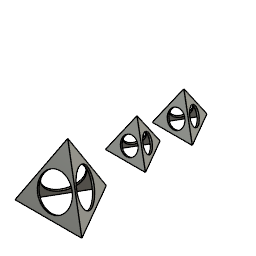
15_DAY- Painter's Tripod (Autodesk Fusion 360 design; units mm, degrees)
part number: 2026-01-01-13-45-42-633
part number: 2026-01-01-14-03-48-325
part number: 2026-01-01-15-44-14-888
part number: 2026-01-01-15-45-19-791
Autodesk Fusion 360 part; units mm, degrees
sketch "Sketch1" plane through (0, 0, 0) normal (0, 1, 0) x (1, 0, 0) in component "60mm Painter's Tripod"
  line L0 (0, 0) -> (30, 51.9615)
  line L1 (30, 51.9615) -> (60, 0)
  line L2 (60, 0) -> (0, 0)
  dimension "d1" = 60
  constraint coincident L0.start L2.end
  constraint horizontal L2
  constraint equal L0 L2
  constraint equal L0 L1
  measures "d1" distance of L0.start L0.end
ref_plane "WorkPlane1" through (30, 50, -25.9808) normal (0, 1, 0) x (1, 0, 0) in component "60mm Painter's Tripod"
sketch "Sketch2" plane through (0, 50, 0) normal (0, 1, 0) x (1, 0, 0) in component "60mm Painter's Tripod"
  line L0 (0, 0) -> (30, 51.9615)
  line L1 (60, 0) -> (0, 0)
  line L2 (30, 51.9615) -> (60, 0)
  line L3 (30, 51.9615) -> (30, 0) construction
  line L4 (0, 0) -> (45, 25.9808) construction
  point P0 (30, 17.3205)
  constraint coincident L0.end L2.start
  constraint midpoint L1 L3.end
  constraint coincident L0.start L1.end
  constraint midpoint L2 L4.end
  constraint coincident L4 P0
  constraint coincident L3 P0
loft "Loft1" add profiles "Sketch1" section 1 section 2 point at (30, 50, -17.3205) makes body 1 in component "60mm Painter's Tripod"
shell "Shell1" thickness 2.5 removed faces 1 at (30, 0, -17.3205) on bodies 1 in component "60mm Painter's Tripod"
sketch "Sketch3" plane through (0, 0, 0) normal (0, 0.327327, 0.944911) x (1, 0, 0) in component "60mm Painter's Tripod"
  line L0 (0, 0) -> (60, 0)
  line L1 (60, 0) -> (30, 52.915)
  line L2 (30, 52.915) -> (0, 0)
  line L3 (30, 52.915) -> (30, 0) construction
  line L4 (0, 0) -> (45, 26.4575) construction
  circle A0 centre (30, 17.6383) radius 12.5
  dimension "d4" = 25
  constraint coincident L1.end L2.start
  constraint midpoint L0 L3.end
  constraint coincident L0.start L2.end
  constraint midpoint L1 L4.end
  constraint coincident L4 A0.centre
  constraint coincident L3 A0.centre
  measures "d4" diameter of A0
extrude "Extrude1" cut sketch "Sketch3" against normal blind 2.5 contours A0 bodies 1 in component "60mm Painter's Tripod"
pattern_circular "C-Pattern1" count 3 over 360 about axis through (30, 75, -17.3205) along (0, -1, 0) of "Extrude1" in component "60mm Painter's Tripod"
sketch "Sketch1 (2)" plane through (0, 0, 0) normal (0, 1, 0) x (1, 0, 0) in component "60mm Painter's Tripod (1)"
  line L0 (0, 0) -> (30, 51.9615)
  line L1 (30, 51.9615) -> (60, 0)
  line L2 (60, 0) -> (0, 0)
  dimension "d1_1" = 60
  constraint coincident L0.start L2.end
  constraint horizontal L2
  constraint equal L0 L2
  constraint equal L0 L1
  measures "d1_1" distance of L0.start L0.end
ref_plane "WorkPlane1" through (30, 50, -25.9808) normal (0, 1, 0) x (1, 0, 0) in component "60mm Painter's Tripod (1)"
sketch "Sketch2 (2)" plane through (0, 50, 0) normal (0, 1, 0) x (1, 0, 0) in component "60mm Painter's Tripod (1)"
  line L0 (0, 0) -> (30, 51.9615)
  line L1 (60, 0) -> (0, 0)
  line L2 (30, 51.9615) -> (60, 0)
  line L3 (30, 51.9615) -> (30, 0) construction
  line L4 (0, 0) -> (45, 25.9808) construction
  point P0 (30, 17.3205)
  constraint coincident L0.end L2.start
  constraint midpoint L1 L3.end
  constraint coincident L0.start L1.end
  constraint midpoint L2 L4.end
  constraint coincident L4 P0
  constraint coincident L3 P0
loft "Loft1'" add profiles "Sketch1 (2)" section 1 section 2 point at (30, 50, -17.3205) separate body makes body 2 in component "60mm Painter's Tripod (1)"
shell "Shell1'" thickness 2.5 removed faces 1 at (30, 0, -17.3205) on bodies 2 in component "60mm Painter's Tripod (1)"
sketch "Sketch3 (2)" plane through (0, 0, 0) normal (0, 0.327327, 0.944911) x (1, 0, 0) in component "60mm Painter's Tripod (1)"
  line L0 (0, 0) -> (60, 0)
  line L1 (60, 0) -> (30, 52.915)
  line L2 (30, 52.915) -> (0, 0)
  line L3 (30, 52.915) -> (30, 0) construction
  line L4 (0, 0) -> (45, 26.4575) construction
  circle A0 centre (30, 17.6383) radius 12.5
  dimension "d4_1" = 25
  constraint coincident L1.end L2.start
  constraint midpoint L0 L3.end
  constraint coincident L0.start L2.end
  constraint midpoint L1 L4.end
  constraint coincident L4 A0.centre
  constraint coincident L3 A0.centre
  measures "d4_1" diameter of A0
extrude "Extrude1'" cut sketch "Sketch3 (2)" against normal blind 2.5 contours A0 bodies 2 in component "60mm Painter's Tripod (1)"
pattern_circular "C-Pattern1'" count 3 over 360 about axis through (30, 75, -17.3205) along (0, -1, 0) of "Extrude1'" in component "60mm Painter's Tripod (1)"
sketch "Sketch1 (3)" plane through (0, 0, 0) normal (0, 1, 0) x (1, 0, 0) in component "60mm Painter's Tripod NEW"
  line L0 (0, 0) -> (50, 86.6025)
  line L1 (50, 86.6025) -> (100, 0)
  line L2 (100, 0) -> (0, 0)
  dimension "d1_2" = 100
  constraint coincident L0.start L2.end
  constraint horizontal L2
  constraint equal L0 L2
  constraint equal L0 L1
  measures "d1_2" distance of L0.start L0.end
ref_plane "WorkPlane1" through (50, 90, -43.3013) normal (0, 1, 0) x (1, 0, 0) in component "60mm Painter's Tripod NEW"
sketch "Sketch2 (3)" plane through (0, 90, 0) normal (0, 1, 0) x (1, 0, 0) in component "60mm Painter's Tripod NEW"
  line L0 (0, 0) -> (50, 86.6025)
  line L1 (100, 0) -> (0, 0)
  line L2 (50, 86.6025) -> (100, 0)
  line L3 (50, 86.6025) -> (50, 0) construction
  line L4 (0, 0) -> (75, 43.3013) construction
  point P0 (50, 28.8675)
  constraint coincident L0.end L2.start
  constraint midpoint L1 L3.end
  constraint coincident L0.start L1.end
  constraint midpoint L2 L4.end
  constraint coincident L4 P0
  constraint coincident L3 P0
loft "Loft1''" add profiles "Sketch1 (3)" section 1 section 2 point at (50, 90, -28.8675) separate body makes body 3 in component "60mm Painter's Tripod NEW"
shell "Shell1''" thickness 2.5 removed faces 1 at (50, 0, -28.8675) on bodies 3 in component "60mm Painter's Tripod NEW"
sketch "Sketch3 (3)" plane through (0, 0, 0) normal (0, 0.305424, 0.952217) x (1, 0, 0) in component "60mm Painter's Tripod NEW"
  line L0 (0, 0) -> (100, 0)
  line L1 (100, 0) -> (50, 94.5163)
  line L2 (50, 94.5163) -> (0, 0)
  line L3 (50, 94.5163) -> (50, 0) construction
  line L4 (0, 0) -> (75, 47.2582) construction
  circle A0 centre (50, 31.5054) radius 25
  dimension "d4_2" = 50
  constraint coincident L1.end L2.start
  constraint midpoint L0 L3.end
  constraint coincident L0.start L2.end
  constraint midpoint L1 L4.end
  constraint coincident L4 A0.centre
  constraint coincident L3 A0.centre
  measures "d4_2" diameter of A0
extrude "Extrude1''" cut sketch "Sketch3 (3)" against normal blind 2.5 contours A0 bodies 3 in component "60mm Painter's Tripod NEW"
pattern_circular "C-Pattern1''" count 3 over 360 about axis through (50, 125, -28.8675) along (0, -1, 0) of "Extrude1''" in component "60mm Painter's Tripod NEW"
component "60mm Painter's Tripod" placed x (1, 0, 0) y (0, 1, 0) z (0, 0, 1) at (0, 0, 0)
component "60mm Painter's Tripod" placed x (1, 0, 0) y (0, 1, 0) z (0, 0, 1) at (0, 0, -70)
component "60mm Painter's Tripod (1)" placed x (1, 0, 0) y (0, 1, 0) z (0, 0, 1) at (0, 0, 0)
component "60mm Painter's Tripod NEW" placed x (1, 0, 0) y (0, 1, 0) z (0, 0, 1) at (0, 0, 0)
